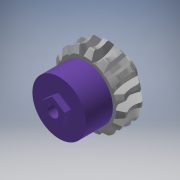
# Autodesk Inventor part: Schneckenrad
Saved by Autodesk Inventor 2019.1 (Build 231200000, 200)
## iProperties
Created: 2018-11-20
Part Number: Schneckenrad
Material: Steel, Mild
Document SubType Name: Modeling
Designer: JochenAlt
Categories: <?xml version="1.0" encoding="UTF-16"?> <MemberInstance><Categories><FamilyTemplate><FamilyTemplateParameter ValueType="xs:double" Id="1" ObjectReferenceKey="da_z" ObjectType="kUserParameterObject"/><FamilyTemplateParameter ValueType="xs:double" Id="2" ObjectReferenceKey="da_b" ObjectType="kUserParameterObject"/><FamilyTemplateParameter ValueType="xs:double" Id="3" ObjectReferenceKey="da_beta" ObjectType="kUserParameterObject"/><FamilyTemplateParameter ValueType="xs:double" Id="4" ObjectReferenceKey="da_m" ObjectType="kUserParameterObject"/><FamilyTemplateParameter ValueType="xs:double" Id="5" ObjectReferenceKey="da_alpha" ObjectType="kUserParameterObject"/><FamilyTemplateParameter ValueType="xs:double" Id="6" ObjectReferenceKey="da_da" ObjectType="kUserParameterObject"/><FamilyTemplateParameter ValueType="xs:double" Id="7" ObjectReferenceKey="da_aw" ObjectType="kUserParameterObject"/><FamilyTemplateParameter ValueType="xs:double" Id="8" ObjectReferenceKey="da_px" ObjectType="kUserParameterObject"/><FamilyTemplateParameter ValueType="xs:double" Id="9" ObjectReferenceKey="da_d" ObjectType="kUserParameterObject"/><FamilyTemplateParameter ValueType="xs:double" Id="10" ObjectReferenceKey="da_dae" ObjectType="kUserParameterObject"/><FamilyTemplateParameter ValueType="xs:double" Id="11" ObjectReferenceKey="da_fi" ObjectType="kUserParameterObject"/><FamilyTemplateParameter ValueType="xs:string" Id="12" ObjectReferenceKey="EAIAABAAAAAWFwAAAAAAAIAAAAAAAAAA" ObjectType="83910656" SubObjectId="SurfaceGeometry"/></FamilyTemplate><ParamToTemplateMap><ParamToTemplate CategoryParameter="//CategoryParameter[@InternalName='046C89C9-8512-4d59-83FE-43B91F4F132A']" TemplateParameter="1"/><ParamToTemplate CategoryParameter="//CategoryParameter[@InternalName='2552DF32-E462-4b46-AEBF-C6C7768E72AC']" TemplateParameter="2"/><ParamToTemplate CategoryParameter="//CategoryParameter[@InternalName='C9EE641D-15FC-4fae-A226-E94C4372FDD7']" TemplateParameter="3"/><ParamToTemplate><ParamToTemplate CategoryParameter="//CategoryParameter[@InternalName='00B6519A-459B-49c7-AD84-2E56D39A5744']" ConstantValue="0.000000"/></ParamToTemplate><ParamToTemplate><ParamToTemplate CategoryParameter="//CategoryParameter[@InternalName='04B31F0E-C7A6-4894-AA32-9629BEFACF47']" ConstantValue="1.000000"/></ParamToTemplate><ParamToTemplate><ParamToTemplate CategoryParameter="//CategoryParameter[@InternalName='43CBEC2E-7847-49e7-A936-2F7889FCB2D9']" ConstantValue="0.200000"/></ParamToTemplate><ParamToTemplate><ParamToTemplate CategoryParameter="//CategoryParameter[@InternalName='B1EFC894-105D-4ebd-86BF-FA20ED196853']" ConstantValue="0.266800"/></ParamToTemplate><ParamToTemplate><ParamToTemplate CategoryParameter="//CategoryParameter[@InternalName='51175063-3D10-4879-93E8-6246FE8B403D']" ConstantValue="2060000000.000000"/></ParamToTemplate><ParamToTemplate><ParamToTemplate CategoryParameter="//CategoryParameter[@InternalName='A3A52E27-4454-46a9-B0BD-C932399B70AF']" ConstantValue="0.300000"/></ParamToTemplate><ParamToTemplate CategoryParameter="//CategoryParameter[@InternalName='91B76062-C214-41d9-B1B9-14D2AB99603D']" TemplateParameter="4"/><ParamToTemplate CategoryParameter="//CategoryParameter[@InternalName='2D373A89-B862-43d6-8D0B-0CBF12AB9F6C']" TemplateParameter="5"/><ParamToTemplate CategoryParameter="//CategoryParameter[@InternalName='37777632-D6A2-4fac-9D53-DB8ACD95C989']" TemplateParameter="6"/><ParamToTemplate CategoryParameter="//CategoryParameter[@InternalName='FD1017F1-B727-4f7e-9707-0F86F1FF9423']" TemplateParameter="7"/><ParamToTemplate CategoryParameter="//CategoryParameter[@InternalName='3BF567DA-17EF-48d8-80EA-D119B07F6463']" TemplateParameter="8"/><ParamToTemplate CategoryParameter="//CategoryParameter[@InternalName='BF5A1E7E-5373-4a22-AAD3-F583781FCF3C']" TemplateParameter="9"/><ParamToTemplate CategoryParameter="//CategoryParameter[@InternalName='2A200944-5A8C-41ca-B96E-8520D2E510F1']" TemplateParameter="10"/><ParamToTemplate CategoryParameter="//CategoryParameter[@InternalName='E77AC4FD-7B43-4566-B0ED-7CA70B976BC8']" TemplateParameter="11"/><ParamToTemplate><ParamToTemplate CategoryParameter="//CategoryParameter[@InternalName='D4F72237-D604-435a-AD0B-F738B7463A00']" ConstantValue="110.000000"/></ParamToTemplate><ParamToTemplate><ParamToTemplate CategoryParameter="//CategoryParameter[@InternalName='9E1B4470-B2D3-4ff1-B813-535BB4CDF51A']" ConstantValue="2000000.000000"/></ParamToTemplate><ParamToTemplate><ParamToTemplate CategoryParameter="//CategoryParameter[@InternalName='A7A89E9A-52E6-4d4f-86CF-A81914F22AA4']" ConstantValue="250000000.000000"/></ParamToTemplate><ParamToTemplate><ParamToTemplate CategoryParameter="//CategoryParameter[@InternalName='B02FABAC-469F-4ad8-A219-DB4578299DF6']" ConstantValue="250000000.000000"/></ParamToTemplate><ParamToTemplate><ParamToTemplate CategoryParameter="//CategoryParameter[@InternalName='E6981962-40D5-4343-A0AD-C263FCC47E10']" ConstantValue="9.000000"/></ParamToTemplate><ParamToTemplate><ParamToTemplate CategoryParameter="//CategoryParameter[@InternalName='B958E99F-2BCD-4955-8634-793EB7B37B89']" ConstantValue="8.000000"/></ParamToTemplate><ParamToTemplate><ParamToTemplate CategoryParameter="//CategoryParameter[@InternalName='4AD49A87-569D-440f-A541-E3B52A6A9DCE']" ConstantValue="1200.000000"/></ParamToTemplate><ParamToTemplate><ParamToTemplate CategoryParameter="//CategoryParameter[@InternalName='4E5813A0-330D-4b41-BE23-D880B01A1D55']" ConstantValue="1650000.000000"/></ParamToTemplate><ParamToTemplate><ParamToTemplate CategoryParameter="//CategoryParameter[@InternalName='19EB8C86-AA88-4253-B4AA-2F5DF1CE171A']" ConstantValue="6000.000000"/></ParamToTemplate><ParamToTemplate CategoryParameter="//CategoryParameter[@InternalName='27C3BAF2-7550-4e4b-AE2C-0DB134B7D9B7']" TemplateParameter="12"/></ParamToTemplateMap><Category DisplayName="Gear" InternalName="DC85795E-93AB-48d5-8EEE-5A27447B64BD" Mnemonic="Gear"><CategoryParameter DisplayName="z" InternalName="046C89C9-8512-4d59-83FE-43B91F4F132A" Mnemonic="z"/><CategoryParameter DisplayName="b|.2|" InternalName="2552DF32-E462-4b46-AEBF-C6C7768E72AC" Mnemonic="b"/><CategoryParameter DisplayName="||b|" InternalName="C9EE641D-15FC-4fae-A226-E94C4372FDD7" Mnemonic="beta"/><CategoryParameter DisplayName="x" InternalName="00B6519A-459B-49c7-AD84-2E56D39A5744" Mnemonic="x"/><CategoryParameter DisplayName="a*" InternalName="04B31F0E-C7A6-4894-AA32-9629BEFACF47" Mnemonic="a"/><CategoryParameter DisplayName="c*" InternalName="43CBEC2E-7847-49e7-A936-2F7889FCB2D9" Mnemonic="c"/><CategoryParameter DisplayName="r|.f|*" InternalName="B1EFC894-105D-4ebd-86BF-FA20ED196853" Mnemonic="rf"/><CategoryParameter DisplayName="E" InternalName="51175063-3D10-4879-93E8-6246FE8B403D" Mnemonic="E"/><CategoryParameter DisplayName="||m|" InternalName="A3A52E27-4454-46a9-B0BD-C932399B70AF" Mnemonic="mi"/><Category DisplayName="WormGear" InternalName="1B25C7EF-093B-4025-B3D3-619CD2A4550C" Mnemonic="WormGear"><CategoryParameter DisplayName="m" InternalName="91B76062-C214-41d9-B1B9-14D2AB99603D" Mnemonic="m"/><CategoryParameter DisplayName="||a|" InternalName="2D373A89-B862-43d6-8D0B-0CBF12AB9F6C" Mnemonic="alpha"/><CategoryParameter DisplayName="d|.a|" InternalName="37777632-D6A2-4fac-9D53-DB8ACD95C989" Mnemonic="da"/><CategoryParameter DisplayName="a|.w|" InternalName="FD1017F1-B727-4f7e-9707-0F86F1FF9423" Mnemonic="aw"/><CategoryParameter DisplayName="p|.x|" InternalName="3BF567DA-17EF-48d8-80EA-D119B07F6463" Mnemonic="px"/><CategoryParameter DisplayName="d" InternalName="BF5A1E7E-5373-4a22-AAD3-F583781FCF3C" Mnemonic="d"/><CategoryParameter DisplayName="dae" InternalName="2A200944-5A8C-41ca-B96E-8520D2E510F1" Mnemonic="dae"/><CategoryParameter DisplayName="||d|" InternalName="E77AC4FD-7B43-4566-B0ED-7CA70B976BC8" Mnemonic="fi"/><CategoryParameter DisplayName="VHV" InternalName="D4F72237-D604-435a-AD0B-F738B7463A00" Mnemonic="VHV"/><CategoryParameter DisplayName="||s||.Hlim|" InternalName="9E1B4470-B2D3-4ff1-B813-535BB4CDF51A" Mnemonic="sHlim"/><CategoryParameter DisplayName="N|.Flim|" InternalName="A7A89E9A-52E6-4d4f-86CF-A81914F22AA4" Mnemonic="NFlim"/><CategoryParameter DisplayName="N|.Hlim|" InternalName="B02FABAC-469F-4ad8-A219-DB4578299DF6" Mnemonic="NHlim"/><CategoryParameter DisplayName="q|.F|" InternalName="E6981962-40D5-4343-A0AD-C263FCC47E10" Mnemonic="qF"/><CategoryParameter DisplayName="q|.H|" InternalName="B958E99F-2BCD-4955-8634-793EB7B37B89" Mnemonic="qH"/><CategoryParameter DisplayName="v|.max|" InternalName="4AD49A87-569D-440f-A541-E3B52A6A9DCE" Mnemonic="maxv"/><CategoryParameter DisplayName="S|.n|" InternalName="4E5813A0-330D-4b41-BE23-D880B01A1D55" Mnemonic="Sn"/><CategoryParameter DisplayName="K|.w|" InternalName="19EB8C86-AA88-4253-B4AA-2F5DF1CE171A" Mnemonic="Kw"/><CategoryParameter DisplayName="PitchDiameter" InternalName="27C3BAF2-7550-4e4b-AE2C-0DB134B7D9B7" Mnemonic="IDS_PITCHDIAM"/></Category></Category></Categories></MemberInstance>
Density: 7.85 g/cm^3
Appearance: Steel
Mass: 32.7133 g
Surface Area: 24.0886 cm^2
Volume: 4.1673 cm^3
CustomPartVersion: 1
Author: JochenAlt
Autodesk Inventor part; units mm, degrees
ref_plane "YZ Plane" through (0, 0, 0) normal (1, 0, 0) x (0, 1, 0)
ref_plane "XZ Plane" through (0, 0, 0) normal (0, 1, 0) x (-1, 0, 0)
ref_plane "XY Plane" through (0, 0, 0) normal (0, 0, 1) x (1, 0, 0)
ref_plane "Zahnebene" through (0, -10, 0) normal (-0.1240347, 0, 0.9922779) x (0, 1, 0)
sketch "Grundkörperskizze" plane through (0, 0, 0) normal (1, 0, 0) x (0, 1, 0)
  line L0 (0, -6.125) -> (0, 6.125) projected
  line L1 (0, 4) -> (9.5727, 4)
  line L2 (9.5727, 4) -> (11.25, 2.6029)
  line L3 (-3.875, 0) -> (23.25, 0) construction
  circle A0 centre (14.375, 0) radius 3.75
  line L4 (11.25, 2.6029) -> (11.25, -2.6029)
  line L5 (0, -4) -> (9.5727, -4)
  line L6 (0, 4) -> (0, -4)
  line L7 (9.5727, -4) -> (11.25, -2.6029)
  dimension "d50" = 39.792
  dimension "d87" = 22.5
  dimension "d89" = 7.5
  dimension "d92" = 8
  dimension "d93" = 14.375
  constraints: 14 end point, 3 symmetric about line, 2 perpendicular, 2 point on line, 1 centre point, 1 collinear
  measures "d50" angle of L2 L1
  measures "d87" diameter of L4 L0
  measures "d89" diameter of A0
  measures "d92" distance of L1.start L5.start
  measures "d93" distance from line of A0.centre L6
revolve "Grundkörper" add sketch "Grundkörperskizze" angle 360 about axis through (0, 0, 0) along (0, 0, 1) picked at (11.1181, -0.4303) contours L0 L1 L2 L4 A0 L7 L5 | A0 L4
revolve "Grundkörper2" cut sketch "Grundkörperskizze" angle 360 about axis through (0, 0, 0) along (0, 0, 1) contours L4 A0 | A0 L4
sketch "Zahnskizze" plane through (0, -10, 0) normal (-0.1240347, 0, 0.9922779) x (0, 1, 0)
  line L0 (10, 2.4137) -> (10, -2.4137) projected
  line L1 (-6.425, 0) -> (3.55, 0) projected
  line L2 (-4.375, 1.7241) -> (-4.375, -1.7241)
  line L3 (-4.375, -1.7241) -> (-0.875, -1.7241)
  line L4 (-0.875, -1.7241) -> (2.125, -0.6321)
  line L5 (2.125, -0.6321) -> (2.125, 0)
  line L6 (2.125, 0.6321) -> (-0.875, 1.7241)
  line L7 (-0.875, 1.7241) -> (-4.375, 1.7241)
  line L8 (2.125, 0.6321) -> (2.125, 0)
  line L9 (0.625, 0) -> (0.625, -1.1781) construction
  dimension "d38" = 14.375
  dimension "d39" = 20
  dimension "d40" = 3.5
  dimension "d41" = 5
  dimension "d42" = 1.1781
  constraints: 16 end point, 4 perpendicular, 3 equal length, 2 point on line, 1 midpoint, 1 parallel, 1 vertical
  measures "d38" distance between parallel lines of L0 L2
  measures "d39" angle of L6 L7
  measures "d40" distance of L6.end L2.start
  measures "d41" distance between parallel lines of L2 L9
  measures "d42" distance of L9.start L9.end
sketch "Sketch8" plane through (0, 0, 4) normal (0, 0, 1) x (1, 0, 0)
  circle A0 centre (0, 0) radius 9.5727 projected
  circle A1 centre (0, 0) radius 9.375
  dimension "d77" = 18.75
  constraints: 1 centre point, 1 coincident
  measures "d77" diameter of A1
surface extrude "Flankendurchmesser" sketch "Sketch8" against normal blind 8 shown no curves A1
ref_plane "Work Plane13" through (0, 0, 0) normal (-0.2079117, 0.9781476, 0) x (0, 0, 1)
revolve "Zahn" cut sketch "Zahnskizze" angle 360 about axis through (-1.7107, -14.375, -0.2138) along (0.9922779, 0, 0.1240347)
pattern_circular "Zahnanordnung" count 15 over 360 about axis through (0, 0, 0) along (0, 0, 1) of "Zahn"
ref_plane "Work Plane14" through (0, 0, 0) normal (0.9781476, 0.2079117, 0) x (0, 0, 1)
ref_plane "Work Plane15" through (0, 0, 0) normal (0, -1, 0) x (0, 0, 1)
sketch "Skizze9" plane through (0, 0, 4) normal (0, 0, 1) x (0.9698388, -0.2437473, 0)
  circle A0 centre (0, 0) radius 1.75
  circle A1 centre (0, 0) radius 4 construction
  line L0 (-4, 0) -> (-1.2361, 3.8042)
  line L1 (-1.2361, 3.8042) -> (3.2361, 2.3511)
  line L2 (3.2361, 2.3511) -> (3.2361, -2.3511)
  line L3 (3.2361, -2.3511) -> (-1.2361, -3.8042)
  line L4 (-1.2361, -3.8042) -> (-4, 0)
  circle A2 centre (0, 0) radius 8.5
  circle A3 centre (0, 0) radius 4.4 construction
  line L5 (-1.3597, 4.1846) -> (3.5597, 2.5863)
  line L6 (3.5597, 2.5863) -> (3.5597, -2.5863)
  line L7 (3.5597, -2.5863) -> (-1.3597, -4.1846)
  line L8 (-1.3597, -4.1846) -> (-4.4, 0)
  line L9 (-4.4, 0) -> (-1.3597, 4.1846)
  dimension "d100" = 8
  dimension "d127" = 0.4
  dimension "d94" = 3.5
  dimension "d101" = 17
  constraints: 20 end point, 6 coincident, 2 centre point, 1 horizontal alignment, 1 parallel, 1 vertical, 27 other
  measures "d94" diameter of A0
  measures "d101" diameter of A2
ref_plane "Arbeitsebene16" through (0, 0, 12.5) normal (0, 0, -1) x (-0.8369419, 0.5472918, 0)
extrude "Extrusion13" add sketch "Skizze9" against normal up to surface (8.5 mm away) from surface at 8.5 separate body contours L0 L1 L2 L3 L4 | A2 | L5 L6 L7 L8 L9
extrude "Extrusion14" add sketch "Skizze9" along normal blind 2 from surface at 8.5 contours L0 L1 L2 L3 L4 bodies 2
extrude "Extrusion15" cut sketch "Skizze9" along normal through all both and the other way through all contours A0 bodies 1 2
sketch "Skizze11" plane through (0, 0, -4) normal (0, 0, -1) x (-0.8369419, 0.5472918, 0)
  circle A0 centre (0, 0) radius 3.35
  circle A1 centre (0, 0) radius 1.75 projected
  circle A2 centre (0, 0) radius 4.35
  dimension "d138" = 6.7
  dimension "d139" = 1
  constraints: 2 centre point, 2 coincident
  measures "d138" diameter of A0
  measures "d139" radial gap between concentric circles of A2 A0
extrude "Extrusion16" add sketch "Skizze11" along normal blind 2 contours A0 | A2 bodies 1
extrude "Extrusion17" add sketch "Skizze11" along normal blind 3 from surface at 2 contours A0 bodies 1
equation "\"d50\" = da_fi"
equation "\"d87\" = da_dae"
equation "\"d89\" = 2 * da_aw - da_da"
equation "\"d92\" = da_b"
equation "\"d93\" = da_aw"
equation "\"d38\" = da_aw"
equation "\"d39\" = da_alfat"
equation "\"d40\" = 0.5 * da_df1"
equation "\"d41\" = 0.5 * da_d1"
equation "\"d42\" = 0.3 * da_px"
equation "\"d77\" = da_dw"
equation "\"d78\" = da_b"
equation "\"da_aw\" = 14.375"
equation "\"da_fi\" = 39.7918deg"
equation "\"da_b\" = 8"
equation "\"da_df\" = 15.75"
equation "\"da_da\" = 21.25"
equation "\"da_beta\" = 7.125016deg"
equation "\"da_alfat\" = 20deg"
equation "\"da_df1\" = 7"
equation "\"da_da1\" = 12.5"
equation "\"da_px\" = 3.926991"
equation "\"d68\" = da_aw"
equation "\"da_dw\" = 18.75"
equation "\"da_rightdir\" = 0"
equation "\"d86\" = da_aw"
equation "\"da_dae\" = 22.5"
equation "\"da_d1\" = 10"
body "Solid1"
body "Srf1"
